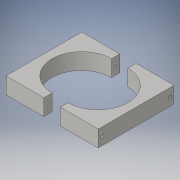
# Autodesk Inventor part: Scuba Tank Holder
Saved by Autodesk Inventor 2016 (Build 200138000, 138)
## iProperties
Created: 2018-05-17
Part Number: Scuba Tank Holder
Material: Generic
Document SubType Name: Modeling
Designer: Kade
Density: 1 g/cm^3
Appearance: Default
Author: Kade
Autodesk Inventor part; units mm, degrees
ref_plane "YZ Plane" through (0, 0, 0) normal (1, 0, 0) x (0, 1, 0)
ref_plane "XZ Plane" through (0, 0, 0) normal (0, 1, 0) x (-1, 0, 0)
ref_plane "XY Plane" through (0, 0, 0) normal (0, 0, 1) x (1, 0, 0)
sketch "Sketch1" plane through (0, 0, 0) normal (0, 1, 0) x (-1, 0, 0)
  line L0 (25.4, -117.408) -> (142.808, -117.408)
  line L1 (142.808, -117.408) -> (142.808, 117.408)
  line L2 (142.808, 117.408) -> (25.4, 117.408)
  line L3 (25.4, 117.408) -> (25.4, 92.008)
  line L4 (25.4, -92.008) -> (25.4, -117.408)
  line L5 (25.4, 117.408) -> (25.4, 92.008)
  line L6 (25.4, -92.008) -> (25.4, -117.408)
  arc A0 (25.4, -92.008) -> (25.4, 92.008) centre (25.4, 0) ccw
  line L7 (-25.4, -117.408) -> (-142.808, -117.408)
  line L8 (-142.808, -117.408) -> (-142.808, 117.408)
  line L9 (-142.808, 117.408) -> (-25.4, 117.408)
  line L10 (-25.4, 117.408) -> (-25.4, 93.412)
  line L11 (-25.4, -92.008) -> (-25.4, -117.408)
  line L12 (-25.4, 117.408) -> (-25.4, 93.412)
  line L13 (-25.4, -92.008) -> (-25.4, -117.408)
  arc A1 (-25.4, 93.412) -> (-25.4, -92.008) centre (-25.4, 0.702) ccw
  point P0 (0, 0)
  dimension "d6" = 25.4
  dimension "d17" = 92.71
  constraints: 28 end point, 4 point on circle, 4 vertical, 3 parallel, 2 centre point, 2 perpendicular
  measures "d6" distance from line of point (0, 0) L4
  measures "d17" radius of A1
extrude "Extrusion1" add sketch "Sketch1" along normal blind 50.8
sketch "Sketch2" plane through (142.808, 0, 117.408) normal (1, 0, 0) x (0, 0, -1)
  circle A0 centre (12.7, 25.4) radius 5.08
  circle A1 centre (225.2508, 25.4) radius 5.08
  circle A2 centre (12.7, 25.4) radius 2.5527
  circle A3 centre (225.2508, 25.4) radius 2.5527
  line L0 (0, 50.8) -> (234.816, 50.8) projected
  line L1 (0, 0) -> (0, 50.8) projected
  point P0 (117.408, 0)
  dimension "d9" = 10.16
  dimension "d10" = 10.16
  dimension "d11" = 5.1054
  dimension "d12" = 5.1054
  dimension "d18" = 25.4
  dimension "d19" = 25.4
  dimension "d21" = 12.7
  constraints: 4 centre point, 2 coincident
  measures "d9" diameter of A0
  measures "d10" diameter of A1
  measures "d11" diameter of A2
  measures "d12" diameter of A3
  measures "d18" distance from line of L0 A0.centre
  measures "d19" distance from line of L0 A1.centre
  measures "d21" distance from line of L1 A0.centre
extrude "Extrusion2" cut sketch "Sketch2" against normal through all contours A2 | A3
extrude "Extrusion3" cut sketch "Sketch2" against normal blind 12.7
body "Solid1"
